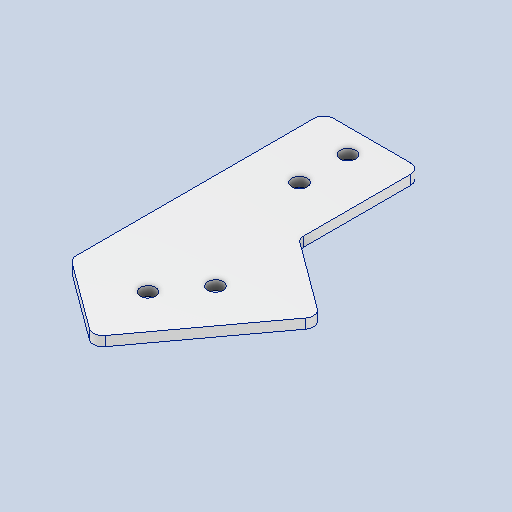
# Autodesk Inventor part: dribl-v3-Plate-13
Saved by Autodesk Inventor 2025.2 (Build 292293000, 293)
## iProperties
Created: 2025-04-05
Part Number: dribl-v3-Plate-13
Material: アルミニウム 6061
Document SubType Name: Modeling
Designer: haruy
Density: 2.7 g/cm^3
Appearance: アルミニウム - フラット
Author: haruy
Autodesk Inventor part; units mm, degrees
ref_plane "YZ Plane" through (0, 0, 0) normal (1, 0, 0) x (0, 1, 0)
ref_plane "XZ Plane" through (0, 0, 0) normal (0, 1, 0) x (-1, 0, 0)
ref_plane "XY Plane" through (0, 0, 0) normal (0, 0, 1) x (1, 0, 0)
derived "dribl-v3-Sketch-Base.ipt"
sketch "スケッチ3" plane through (400, -212.3334, -323) normal (0, 1, 0) x (1, 0, 0)
  circle A0 centre (-300, 150) radius 360 projected
  line L0 (-20, 84.0011) -> (-20, 318.8333) projected
  line L1 (0, -20) -> (-20, -20) projected
  line L2 (-255, -130) -> (-275, -130) projected
  line L3 (-275, -130) -> (-275, 430) projected
  line L4 (-275, 430) -> (-255, 430) projected
  line L5 (-255, 430) -> (-255, -130) projected
  line L6 (-325, -130) -> (-345, -130) projected
  line L7 (-345, -130) -> (-345, 430) projected
  line L8 (-345, 430) -> (-325, 430) projected
  line L9 (-325, 430) -> (-325, -130) projected
  line L10 (-600, 450) -> (0, 450) projected
  line L11 (0, 450) -> (0, -150) projected
  line L12 (0, -150) -> (-600, -150) projected
  line L13 (-600, -150) -> (-600, 450) projected
  line L14 (-600, 450) -> (0, -150) construction
  line L15 (0, 450) -> (-600, -150) construction
  line L16 (-130, -150) -> (-470, -150) projected
  line L17 (-470, -150) -> (-470, -130) projected
  line L18 (-470, -130) -> (-130, -130) projected
  line L19 (-130, -130) -> (-130, -150) projected
  line L20 (-300, 150) -> (-660, 150) projected
  line L21 (-130, 450) -> (-470, 450) projected
  line L22 (-130, 430) -> (-130, 450) projected
  line L23 (-470, 430) -> (-130, 430) projected
  line L24 (-470, 450) -> (-470, 430) projected
  line L25 (0, 0) -> (-20, 0) projected
  line L26 (-20, 0) -> (-20, 255) projected
  line L27 (-20, 255) -> (0, 255) projected
  line L28 (0, 255) -> (0, 0) projected
  line L29 (0, 60) -> (-20, 60) projected
  line L30 (-580, 0) -> (-20, 0) projected
  line L31 (0, 230) -> (-20, 230) projected
  line L32 (-21.7796, 57.5848) -> (-158.2154, -127.578) projected
  line L33 (-158.2154, -127.578) -> (-174.3165, -115.714) projected
  line L34 (-174.3165, -115.714) -> (-37.8807, 69.4488) projected
  line L35 (-37.8807, 69.4488) -> (-21.7796, 57.5848) projected
  line L36 (-300, 150) -> (-300, -130) projected
  line L37 (-160, -150) -> (-160, -130) projected
  line L38 (-160, -130) -> (-20, 60) projected
  line L39 (-160, 430) -> (-160, 450) projected
  line L40 (-160, 430) -> (-20, 230) projected
  line L41 (-24.5877, 236.5539) -> (-156.484, 424.9772) projected
  line L42 (-156.484, 424.9772) -> (-172.8687, 413.508) projected
  line L43 (-172.8687, 413.508) -> (-40.9723, 225.0846) projected
  line L44 (-40.9723, 225.0846) -> (-24.5877, 236.5539) projected
  line L45 (-427.1313, 413.508) -> (-559.0277, 225.0846) projected
  line L46 (-575.4123, 236.5539) -> (-443.516, 424.9772) projected
  line L47 (-443.516, 424.9772) -> (-427.1313, 413.508) projected
  line L48 (-559.0277, 225.0846) -> (-575.4123, 236.5539) projected
  line L49 (-562.1193, 69.4488) -> (-578.2204, 57.5848) projected
  line L50 (-578.2204, 57.5848) -> (-441.7846, -127.578) projected
  line L51 (-425.6835, -115.714) -> (-562.1193, 69.4488) projected
  line L52 (-441.7846, -127.578) -> (-425.6835, -115.714) projected
  line L53 (-130, -150) -> (-150, -150) projected
  line L54 (-150, -150) -> (-150, -130) projected
  line L55 (-150, -130) -> (-130, -130) projected
  line L56 (-130, -130) -> (-130, -150) projected
  line L57 (-470, -130) -> (-450, -130) projected
  line L58 (-450, -130) -> (-450, -150) projected
  line L59 (-450, -150) -> (-470, -150) projected
  line L60 (-470, -150) -> (-470, -130) projected
  line L61 (-130, 450) -> (-150, 450) projected
  line L62 (-150, 450) -> (-150, 430) projected
  line L63 (-150, 430) -> (-130, 430) projected
  line L64 (-130, 430) -> (-130, 450) projected
  line L65 (-470, 450) -> (-450, 450) projected
  line L66 (-450, 450) -> (-450, 430) projected
  line L67 (-450, 430) -> (-470, 430) projected
  line L68 (-470, 430) -> (-470, 450) projected
  line L69 (-255, 150) -> (-345, 150) projected
  line L70 (-156.484, 424.9772) -> (-160, 430) projected
  circle A1 centre (-165, 440) radius 1.6 projected
  circle A2 centre (-175, 440) radius 1.6 projected
  line L71 (-172.8687, 413.508) -> (-184.4131, 430) projected
  line L72 (-184.4131, 430) -> (-184.4131, 450) projected
  circle A3 centre (-161.809, 415.1464) radius 1.6 projected
  circle A4 centre (-156.0744, 406.9541) radius 1.6 projected
  circle A5 centre (-425, 440) radius 1.6 projected
  circle A6 centre (-435, 440) radius 1.6 projected
  circle A7 centre (-438.191, 415.1464) radius 1.6 projected
  circle A8 centre (-443.9256, 406.9541) radius 1.6 projected
  circle A9 centre (-435, -140) radius 1.6 projected
  circle A10 centre (-425, -140) radius 1.6 projected
  circle A11 centre (-175, -140) radius 1.6 projected
  circle A12 centre (-165, -140) radius 1.6 projected
  circle A13 centre (-10, 225) radius 1.6 projected
  circle A14 centre (-10, 205) radius 1.6 projected
  circle A15 centre (-35.6473, 234.9154) radius 1.6 projected
  circle A16 centre (-41.382, 243.1077) radius 1.6 projected
  line L73 (-36.0569, 252.9385) -> (-52.4416, 241.4692) projected
  line L74 (-40.9723, 225.0846) -> (-20, 195.1241) projected
  line L75 (-20, 195.1241) -> (0, 195.1241) projected
  circle A17 centre (-558.618, 243.1077) radius 1.6 projected
  circle A18 centre (-564.3527, 234.9154) radius 1.6 projected
  circle A19 centre (-590, 225) radius 1.6 projected
  circle A20 centre (-590, 205) radius 1.6 projected
  line L76 (-37.8807, 69.4488) -> (-20, 93.7155) projected
  circle A21 centre (-10, 65) radius 1.6 projected
  circle A22 centre (-10, 85) radius 1.6 projected
  line L77 (-20, 93.7155) -> (0, 93.7155) projected
  circle A23 centre (-32.7962, 59.4915) radius 1.6 projected
  circle A24 centre (-38.7281, 51.441) radius 1.6 projected
  line L78 (-33.6436, 41.4837) -> (-49.7447, 53.3477) projected
  circle A25 centre (-590, 65) radius 1.6 projected
  circle A26 centre (-590, 85) radius 1.6 projected
  circle A27 centre (-567.2038, 59.4915) radius 1.6 projected
  circle A28 centre (-561.2719, 51.441) radius 1.6 projected
  circle A29 centre (-265, 420) radius 1.6 projected
  circle A30 centre (-265, 410) radius 1.6 projected
  circle A31 centre (-265, 440) radius 1.6 projected
  circle A32 centre (-255, 440) radius 1.6 projected
  line L79 (-250, 430) -> (-250, 450) projected
  line L80 (-255, 405) -> (-275, 405) projected
  circle A33 centre (-335, 440) radius 1.6 projected
  circle A34 centre (-345, 440) radius 1.6 projected
  circle A35 centre (-335, 420) radius 1.6 projected
  circle A36 centre (-335, 410) radius 1.6 projected
  circle A37 centre (-345, -140) radius 1.6 projected
  circle A38 centre (-335, -140) radius 1.6 projected
  circle A39 centre (-335, -120) radius 1.6 projected
  circle A40 centre (-335, -110) radius 1.6 projected
  circle A41 centre (-265, -140) radius 1.6 projected
  circle A42 centre (-255, -140) radius 1.6 projected
  circle A43 centre (-265, -120) radius 1.6 projected
  circle A44 centre (-265, -110) radius 1.6 projected
  line L81 (-74.2, 10) -> (-125, 10) projected
  line L82 (-125, 10) -> (-125, 317) projected
  line L83 (-125, 317) -> (-74.2, 317) projected
  line L84 (-74.2, 317) -> (-74.2, 10) projected
  line L85 (-125, 44.5) -> (-105, 44.5) projected
  line L86 (-105, 44.5) -> (-105, 59.5) projected
  line L87 (-105, 59.5) -> (-125, 59.5) projected
  line L88 (-125, 59.5) -> (-125, 44.5) projected
  line L89 (-125, 163.5) -> (-74.2, 163.5) projected
  line L90 (-105, 282.5) -> (-105, 267.5) projected
  line L91 (-125, 282.5) -> (-105, 282.5) projected
  line L92 (-105, 267.5) -> (-125, 267.5) projected
  line L93 (-125, -16.5) -> (-105, -16.5) projected
  line L94 (-105, -16.5) -> (-105, 313.5) projected
  line L95 (-105, 313.5) -> (-125, 313.5) projected
  line L96 (-125, 313.5) -> (-125, -16.5) projected
  circle A45 centre (-115, -1.5) radius 1.6 projected
  circle A46 centre (-115, -11.5) radius 1.6 projected
  line L97 (-125, 3.5) -> (-105, 3.5) projected
  line L98 (-125, -16.5) -> (-125, -48.7845) projected
  line L99 (-125, -48.7845) -> (-108.8989, -60.6485) projected
  circle A47 centre (-111.0984, -46.7758) radius 1.6 projected
  circle A48 centre (-105.1664, -38.7253) radius 1.6 projected
  circle A49 centre (-115, 298.5) radius 1.6 projected
  circle A50 centre (-115, 308.5) radius 1.6 projected
  line L100 (-125, 293.5) -> (-105, 293.5) projected
  line L101 (-125, 313.5) -> (-125, 345.1241) projected
  line L102 (-105, 313.5) -> (-105, 316.5527) projected
  line L103 (-105, 316.5527) -> (-88.6154, 328.0219) projected
  circle A51 centre (-102.7424, 330.7655) radius 1.6 projected
  circle A52 centre (-108.477, 338.9578) radius 1.6 projected
  line L104 (-125, 345.1241) -> (-108.6154, 356.5934) projected
  line L105 (-105, -16.5) -> (-105, -21.6416) projected
  line L106 (-105, -21.6416) -> (-88.8989, -33.5056) projected
  circle A53 centre (-160.3339, -113.5955) radius 1.5 projected
  circle A54 centre (-154.402, -105.5449) radius 1.5 projected
  circle A55 centre (-439.6661, -113.5955) radius 1.5 projected
  circle A56 centre (-445.598, -105.5449) radius 1.5 projected
  point P0 (-400, -323)
  point P1 (-265, 120)
  point P2 (-335, 120)
  point P3 (-265, 270)
  point P4 (-335, 270)
  point P5 (-99.6, 163.5)
  point P6 (-108.8989, -60.6485)
  point P7 (-88.8989, -33.5056)
  constraints: 1 horizontal alignment
extrude "押し出し1" add sketch "スケッチ3" along normal blind 2 contours L32 L99 L34 L106 | L94 L93 L96 L30 A45 | L30 A45 L96 L97 L94 | L34 L98 L93 L105
fillet "フィレット1" radius 2 6 edges at (295, -211.3334, -326.5) (275, -211.3334, -326.5) (295, -211.3334, -301.3584) (311.1011, -211.3334, -289.4944) (291.1011, -211.3334, -262.3515) (275, -211.3334, -274.2155)
